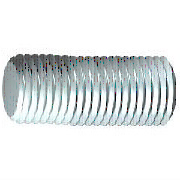
# Autodesk Inventor part: DIN 976-1 - M16 x 1,5 x 240 - A
Saved by Autodesk Inventor 2023 (Build 270158000, 158)
## iProperties
Created: 2022-02-04
Part Number: DIN 976-1 - M16 x 1,5 x 240 - A
Material: Сталь, мягкая
Description: Шпильки с резьбой по всей длине - часть 1: метрическая резьба
Document SubType Name: Modeling
Standard: DIN 976-1
Designer: stepa
Standard Revision: 2002-12
Standards Organization: DIN
Language: ru-RU
Size Designation: M16 x 1,5 x 240
Categories: <MemberInstance><Categories><Category DisplayName="Крепежные изделия" InternalName="e4da775c-781d-43d5-af7c-5136215cf5a6" Mnemonic="FSTN"><Category DisplayName="Болты  Винты" InternalName="536e6df0-f778-49ac-b2f2-25c71d2aa0b2" Mnemonic="SCRW"><CategoryParameter DisplayName="Обозначение номинального диаметра" InternalName="03caf894-eafd-4c09-a035-916ac084b87b" Mnemonic="nomdiadesig"/><CategoryParameter DisplayName="Номинальная длина" InternalName="238ecbaf-3e6c-45dd-aa95-4068c8e0fd02" Mnemonic="nomlen"/><CategoryParameter DisplayName="Обозначение резьбы" InternalName="586d5e89-370a-4089-914f-0110033585c7" Mnemonic="thrdesign"/><CategoryParameter DisplayName="Обозначение серии резьб" InternalName="87c5849c-b3a5-4c3e-9c9b-2feecef9be86" Mnemonic="thrserdsgn"/><CategoryParameter DisplayName="Номинальный диаметр" InternalName="8bbe3f8e-44cf-40a9-a251-3a6edc8168d6" Mnemonic="nomdia"/><CategoryParameter DisplayName="Тип резьбы" InternalName="b4bbb7bc-d6aa-4c9f-a9a9-4152b9f6fe49" Mnemonic="thrtype"/><CategoryParameter DisplayName="Шаг резьбы" InternalName="bb82302e-82d8-4176-8fc1-c5d7bb17d5ad" Mnemonic="pitch1"/><CategoryParameter DisplayName="Витков на единицу" InternalName="bdc6e7d2-ffd0-4d9c-a173-16b95ebb912d" Mnemonic="thrperunit1"/><CategoryParameter DisplayName="Класс резьбы" InternalName="ebc0d23b-2cc6-4d2a-b376-d52aae53bab6" Mnemonic="thrclss"/><Category DisplayName="Шпильки" InternalName="f271271b-2709-4fa4-9e00-74345d22d1b9" Mnemonic="STSCRW"><CategoryParameter DisplayName="Длина резьбы" InternalName="44120fa9-458c-4afd-b05d-4f0a9e7c8b12" Mnemonic="thrlen"/><CategoryParameter DisplayName="Диаметр стержня" InternalName="5c626369-b708-4d6f-96f0-6ba8b9bec5e7" Mnemonic="grpdia"/><CategoryParameter DisplayName="Длина второй резьбы" InternalName="96256c40-12d1-4e29-8396-4efe0ad991a1" Mnemonic="thrlen2"/><CategoryParameter DisplayName="Длина стержня" InternalName="c59dacd6-ffb6-4176-bb92-c0b02633de53" Mnemonic="grplen"/><CategoryParameter DisplayName="Тип" InternalName="f0ad756d-6243-457b-878f-d1d10eeb6a5f" Mnemonic="type"/></Category></Category></Category><Category DisplayName="ТипДанных" InternalName="23b78d0f-2648-40c6-8793-ca6db495c9e8" Mnemonic="DATATYPE"><CategoryParameter DisplayName="ОтображаемоеИмя" InternalName="05415f3d-3907-474b-a020-eb9d644f4cf3" Mnemonic="DISPLAYNAME"/><CategoryParameter DisplayName="Стандарт" InternalName="0c0a119c-1e12-4c84-803f-101930972f5e" Mnemonic="STANDARD"/><CategoryParameter DisplayName="Наименование" InternalName="13903e3d-64b1-4950-80da-f627842ea37f" Mnemonic="DESCRIPTION"/><CategoryParameter DisplayName="Обозначение" InternalName="2675968c-4ce5-49e0-a4f5-552d29089031" Mnemonic="DESIGNATION"/><CategoryParameter DisplayName="Строка по умолчанию" InternalName="2af9ec52-faaa-4026-b378-f9fa4afca842" Mnemonic="DEFAULTROW"/><CategoryParameter DisplayName="Имя папки" InternalName="3f06958e-8713-4116-9be7-ed6184ecc97b" Mnemonic="FOLDERNAME"/><CategoryParameter DisplayName="Указатель редакций" InternalName="45a75005-10b1-4dfc-8d6d-dfe629f0b93c" Mnemonic="REVISIONGUID"/><CategoryParameter DisplayName="ИмяФайла" InternalName="8b46a4cc-9585-4fed-90c3-899f57e09a73" Mnemonic="FILENAME"/><CategoryParameter DisplayName="ОргСтанд" InternalName="8f5914e1-4693-403f-8ab5-d37768198c9d" Mnemonic="STDSORG"/><CategoryParameter DisplayName="Версия семейства" InternalName="914462f6-6e19-4b14-ba84-155b9680b1d0" Mnemonic="FAMILYREVISION"/><CategoryParameter DisplayName="Редакция стандарта" InternalName="91d5a463-65c2-4fde-b823-3b7fea5e8e17" Mnemonic="STANDARDREVISION"/><CategoryParameter DisplayName="редакция элемента" InternalName="a65d44b9-392f-4f4f-857b-e4b3d54996fe" Mnemonic="MEMBERREVISION"/><CategoryParameter DisplayName="ФорматКлипа" InternalName="bc51e27b-3422-4e78-93ef-cec197ddf230" Mnemonic="CLIPFORMAT"/><CategoryParameter DisplayName="Изготовитель" InternalName="cd6c7a72-a28a-4e50-99a9-2c7f4e13e5ad" Mnemonic="MANUFACTURER"/><CategoryParameter DisplayName="ВнутреннееИмя" InternalName="cf1d0246-76d9-4b4a-8305-fa0409afb5c1" Mnemonic="INTERNALNAME"/><CategoryParameter DisplayName="Метрическая" InternalName="e2385c5b-1ea4-4823-96a8-8de651266ec3" Mnemonic="ISMETRIC"/><Category DisplayName="Деталь" InternalName="c0e0b642-3bcb-4cc8-9e80-f96d35c4afa4" Mnemonic="PART"><CategoryParameter DisplayName="Номер детали" InternalName="016b6077-bfbe-49bd-92c9-d8d59c39c941" Mnemonic="PARTNUMBER"/><CategoryParameter DisplayName="Инвентарный номер" InternalName="4dba7c1c-e26c-444e-836c-b08b433409a8" Mnemonic="STOCKNUMBER"/><CategoryParameter DisplayName="Ключ материала" InternalName="5c9a8adb-dd2b-4535-b97f-0a94a95fe41f" Mnemonic="MATERIALKEY"/><CategoryParameter DisplayName="Материал" InternalName="818a152a-d3c3-49ca-80ee-df7d91421b8e" Mnemonic="MATERIAL"/></Category></Category><Category DisplayName="СтараяКарта" InternalName="cd87c42b-3e48-431e-b5c0-1cbeb14dfe77" Mnemonic="LEGACYMAP"><CategoryParameter DisplayName="уникальное обозначение элемента DA" InternalName="0918ad47-427f-4fed-ae26-24c81c58f590" Mnemonic="DACOOKIE"/><CategoryParameter DisplayName="Объединить код 11" InternalName="0ee8fb18-e2ed-4f39-96f6-1f4b5f50aa71" Mnemonic="MERGE11"/><CategoryParameter DisplayName="уникальное обозначение элемента CC" InternalName="5193edd4-b2b0-4ab4-9d54-de900eee34e0" Mnemonic="CCCOOKIE"/><CategoryParameter DisplayName="Разделить код" InternalName="72b5c83c-be7f-45c4-ae51-9160ea6deb26" Mnemonic="SPLIT"/><CategoryParameter DisplayName="КодУчастника" InternalName="8e5e0294-fc51-4c8f-b3d7-003dc5ed94f6" Mnemonic="MEMBERID"/><CategoryParameter DisplayName="ИмяКаталога" InternalName="d99d1e27-aa94-4de2-af4c-c348882a6f4f" Mnemonic="CATALOGNAME"/><CategoryParameter DisplayName="НомерСемейства" InternalName="e705e1f4-09cb-413e-91f9-551b4188271e" Mnemonic="FAMILYNUMBER"/></Category></Categories><FamilyTemplate Id="D976-1A"><FamilyTemplateParameters><FamilyTemplateParameter ObjectType="kUserParameterObject" ValueType="xs:double" Id="1" ObjectReferenceKey="GUL"/><FamilyTemplateParameter ObjectType="kUserParameterObject" ValueType="xs:double" Id="2" ObjectReferenceKey="SPD"/><FamilyTemplateParameter ObjectType="kUserParameterObject" ValueType="xs:double" Id="3" ObjectReferenceKey="TPU"/><FamilyTemplateParameter ObjectType="kUserParameterObject" ValueType="xs:double" Id="4" ObjectReferenceKey="PTC"/><FamilyTemplateParameter ObjectType="kUserParameterObject" ValueType="xs:double" Id="5" ObjectReferenceKey="GEL"/><FamilyTemplateParameter ObjectType="kUserParameterObject" ValueType="xs:double" Id="6" ObjectReferenceKey="THREADDIA"/><FamilyTemplateParameter ObjectType="kUserParameterObject" ValueType="xs:double" Id="7" ObjectReferenceKey="TOA"/><FamilyTemplateParameter ObjectType="kUserParameterObject" ValueType="xs:double" Id="9" ObjectReferenceKey="NLG"/><FamilyTemplateParameter ObjectType="kUserParameterObject" ValueType="xs:double" Id="11" ObjectReferenceKey="GUL1"/><FamilyTemplateParameter ObjectType="kUserParameterObject" ValueType="xs:double" Id="12" ObjectReferenceKey="NND"/><FamilyTemplateParameter ObjectType="kUserParameterObject" ValueType="xs:double" Id="13" ObjectReferenceKey="GAL1"/><FamilyTemplateParameter ObjectType="kUserParameterObject" ValueType="xs:double" Id="15" ObjectReferenceKey="GAL"/><FamilyTemplateParameter ObjectType="kUserParameterObject" ValueType="xs:double" Id="16" ObjectReferenceKey="GD1"/><FamilyTemplateParameter ObjectType="kPropertyObject" ValueType="xs:string" Id="100" ObjectReferenceKey="{32853F0F-3444-11d1-9E93-0060B03C1CA6}" SubObjectId="52"/><FamilyTemplateParameter ObjectType="kPropertyObject" ValueType="xs:string" Id="105" ObjectReferenceKey="{32853F0F-3444-11d1-9E93-0060B03C1CA6}" SubObjectId="5"/><FamilyTemplateParameter ObjectType="kPartComponentDefinitionObject" ValueType="xs:string" Id="110" SubObjectId="Material"/><FamilyTemplateParameter ObjectType="kThreadFeatureObject" ValueType="xs:structure" Id="300" ObjectReferenceKey="1002000010000000e8010000000000008000000000000000" SubObjectId="ThreadInfo"><FamilyTemplateParameter ObjectType="" ValueType="xs:string" Id="301" SubObjectId="ThreadDesignation"/><FamilyTemplateParameter ObjectType="" ValueType="xs:string" Id="302" SubObjectId="ThreadType"/><FamilyTemplateParameter ObjectType="" ValueType="xs:string" Id="303" SubObjectId="ThreadClass"/></FamilyTemplateParameter></FamilyTemplateParameters></FamilyTemplate><CategoryParameterMap><ParamToTemplateMap><ParamToTemplate CategoryParameter="//CategoryParameter[@InternalName='05415f3d-3907-474b-a020-eb9d644f4cf3']" ConstantValue="DIN 976-1 A"/><ParamToTemplate CategoryParameter="//CategoryParameter[@InternalName='cf1d0246-76d9-4b4a-8305-fa0409afb5c1']" ConstantValue="4DDA4BDF-3952-4EE6-BE5D-51A74CFA4C58"/><ParamToTemplate CategoryParameter="//CategoryParameter[@InternalName='3f06958e-8713-4116-9be7-ed6184ecc97b']" ConstantValue="DIN 976-1 A"/><ParamToTemplate CategoryParameter="//CategoryParameter[@InternalName='914462f6-6e19-4b14-ba84-155b9680b1d0']" ConstantValue="10"/><ParamToTemplate CategoryParameter="//CategoryParameter[@InternalName='bc51e27b-3422-4e78-93ef-cec197ddf230']" ConstantValue="CF_INVENTOR.STDPARTS"/><ParamToTemplate CategoryParameter="//CategoryParameter[@InternalName='e2385c5b-1ea4-4823-96a8-8de651266ec3']" ConstantValue="true"/><ParamToTemplate CategoryParameter="//CategoryParameter[@InternalName='13903e3d-64b1-4950-80da-f627842ea37f']" ConstantValue="Stud bolts - Part 1: Metric thread"/><ParamToTemplate CategoryParameter="//CategoryParameter[@InternalName='8f5914e1-4693-403f-8ab5-d37768198c9d']" ConstantValue="DIN"/><ParamToTemplate CategoryParameter="//CategoryParameter[@InternalName='0c0a119c-1e12-4c84-803f-101930972f5e']" ConstantValue="DIN 976-1"/><ParamToTemplate CategoryParameter="//CategoryParameter[@InternalName='cd6c7a72-a28a-4e50-99a9-2c7f4e13e5ad']" TemplateParameter="104"/><ParamToTemplate CategoryParameter="//CategoryParameter[@InternalName='91d5a463-65c2-4fde-b823-3b7fea5e8e17']" ConstantValue="2002-12"/><ParamToTemplate CategoryParameter="//CategoryParameter[@InternalName='45a75005-10b1-4dfc-8d6d-dfe629f0b93c']" ConstantValue="08edc590-c8cc-4f64-a033-9cdc555b26e7"/><ParamToTemplate CategoryParameter="//CategoryParameter[@InternalName='2af9ec52-faaa-4026-b378-f9fa4afca842']" ConstantValue="10"/><ParamToTemplate CategoryParameter="//CategoryParameter[@InternalName='d99d1e27-aa94-4de2-af4c-c348882a6f4f']" ConstantValue="DIN"/><ParamToTemplate CategoryParameter="//CategoryParameter[@InternalName='e705e1f4-09cb-413e-91f9-551b4188271e']" ConstantValue="9761"/><ParamToTemplate CategoryParameter="//CategoryParameter[@InternalName='8b46a4cc-9585-4fed-90c3-899f57e09a73']" ConstantValue="DIN 976-1 - M16 x 1,5 x 240 - A"/><ParamToTemplate CategoryParameter="//CategoryParameter[@InternalName='a65d44b9-392f-4f4f-857b-e4b3d54996fe']" ConstantValue="391AA8AE-0837-4227-BC01-4CC4335BD765"/><ParamToTemplate CategoryParameter="//CategoryParameter[@InternalName='ebc0d23b-2cc6-4d2a-b376-d52aae53bab6']" ConstantValue="6g"/><ParamToTemplate CategoryParameter="//CategoryParameter[@InternalName='03caf894-eafd-4c09-a035-916ac084b87b']" ConstantValue="M16 x 1.5"/><ParamToTemplate CategoryParameter="//CategoryParameter[@InternalName='b4bbb7bc-d6aa-4c9f-a9a9-4152b9f6fe49']" ConstantValue="ISO Metric profile"/><ParamToTemplate CategoryParameter="//CategoryParameter[@InternalName='8e5e0294-fc51-4c8f-b3d7-003dc5ed94f6']" ConstantValue="5370"/><ParamToTemplate CategoryParameter="//CategoryParameter[@InternalName='2675968c-4ce5-49e0-a4f5-552d29089031']" TemplateParameter="100"/><ParamToTemplate CategoryParameter="//CategoryParameter[@InternalName='44120fa9-458c-4afd-b05d-4f0a9e7c8b12']" TemplateParameter="5"/><ParamToTemplate CategoryParameter="//CategoryParameter[@InternalName='818a152a-d3c3-49ca-80ee-df7d91421b8e']" TemplateParameter="110"/><ParamToTemplate CategoryParameter="//CategoryParameter[@InternalName='238ecbaf-3e6c-45dd-aa95-4068c8e0fd02']" TemplateParameter="9"/><ParamToTemplate CategoryParameter="//CategoryParameter[@InternalName='8bbe3f8e-44cf-40a9-a251-3a6edc8168d6']" TemplateParameter="12"/><ParamToTemplate CategoryParameter="//CategoryParameter[@InternalName='016b6077-bfbe-49bd-92c9-d8d59c39c941']" TemplateParameter="105"/><ParamToTemplate CategoryParameter="//CategoryParameter[@InternalName='bb82302e-82d8-4176-8fc1-c5d7bb17d5ad']" TemplateParameter="4"/><ParamToTemplate CategoryParameter="//CategoryParameter[@InternalName='586d5e89-370a-4089-914f-0110033585c7']" TemplateParameter="301"/><ParamToTemplate CategoryParameter="//CategoryParameter[@InternalName='bdc6e7d2-ffd0-4d9c-a173-16b95ebb912d']" TemplateParameter="3"/></ParamToTemplateMap></CategoryParameterMap></MemberInstance>
Density: 7.85 g/cm^3
Appearance: С умеренной полировкой
IsCustomPart: 0
Author: stepa
Autodesk Inventor part; units mm, degrees
ref_plane "YZ Plane" through (0, 0, 0) normal (1, 0, 0) x (0, 1, 0)
ref_plane "XZ Plane" through (0, 0, 0) normal (0, 1, 0) x (-1, 0, 0)
sketch "Эскиз1" plane through (0, 0, 0) normal (0, 0, 1) x (1, 0, 0)
  line L0 (120, 8) -> (120, 0)
  line L1 (-120, 0) -> (120, 0)
  line L2 (-168, 0) -> (168, 0) projected
  line L3 (0, 9.6) -> (0, -1.6) projected
  line L4 (-120, 8) -> (-120, 0)
  line L5 (0, 8) -> (0, 0) construction
  line L6 (-168, 0) -> (168, 0) projected
  line L7 (-120, 8) -> (120, 8)
  dimension "d13" = 16
  dimension "d87" = 240
  dimension "d88" = 120
  constraints: 10 end point, 3 perpendicular, 2 midpoint, 1 parallel, 1 point on line
  measures "d13" diameter of L7 L1
  measures "d87" distance between parallel lines of L4 L0
  measures "d88" distance between parallel lines of L3 L0
revolve "Базовый элемент" add sketch "Эскиз1" angle 360 about axis through (-120, 0, 0) along (1, 0, 0)
thread "Резьба1" size "M16x1.5" class "6g" standard "ISO Metric profile" length 240
ref_plane "Work Plane1" through (2.75, 0, 0) normal (0, -1, 0) x (1, 0, 0)
equation "\"d13\" = NND"
equation "\"d87\" = NLG"
equation "\"d88\" = 0.5 * NLG"
equation "\"d1\" = GEL"
equation "\"NLG\" = 240"
equation "\"GEL\" = NLG"
equation "\"GAL\" = 0.61345 * PTC"
equation "\"SPD\" = 13.93"
equation "\"d0\" = NND"
equation "\"GUL\" = 0.61345 * PTC"
equation "\"NND\" = 16"
equation "\"GUL1\" = GUL"
equation "\"GAL1\" = GAL"
equation "\"d89\" = -GEL + GUL1"
equation "\"d90\" = -GUL - GEL"
equation "\"PTC\" = 1.5"
equation "\"THREADDIA\" = 16"
equation "\"TOA\" = 30deg"
equation "\"GD1\" = THREADDIA - 1.2269 * PTC"
body "Solid1"
